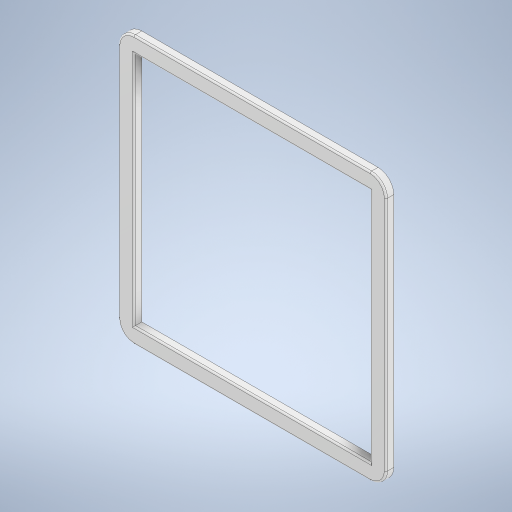
# Autodesk Inventor part: frame_inner
Saved by Autodesk Inventor 2023 (Build 270158000, 158)
## iProperties
Created: 2022-11-05
Part Number: frame_inner
Material: Acetalharz, Weiß
Document SubType Name: Modeling
Designer: RubenStein
Density: 1.425 g/cm^3
Appearance: Glatt - Weiß
Mass: 44.9884 g
Surface Area: 189.425 cm^2
Volume: 31.5708 cm^3
Author: RubenStein
Autodesk Inventor part; units mm, degrees
ref_plane "YZ Plane" through (0, 0, 0) normal (1, 0, 0) x (0, 1, 0)
ref_plane "XZ Plane" through (0, 0, 0) normal (0, 1, 0) x (-1, 0, 0)
ref_plane "XY Plane" through (0, 0, 0) normal (0, 0, 1) x (1, 0, 0)
sketch "Skizze1" plane through (0, 0, 0) normal (0, 0, 1) x (1, 0, 0)
  line L0 (0, 0) -> (170, 0)
  line L1 (170, 0) -> (170, 170)
  line L2 (170, 170) -> (0, 170)
  line L3 (0, 170) -> (0, 0)
  line L4 (10, 10) -> (160, 10)
  line L5 (160, 10) -> (160, 160)
  line L6 (160, 160) -> (10, 160)
  line L7 (10, 160) -> (10, 10)
  dimension "d0" = 170
  dimension "d1" = 10
  dimension "d2" = 10
  dimension "d3" = 150
  constraints: 16 end point, 4 parallel, 4 perpendicular, 2 horizontal
  measures "d0" distance of L1.end L2.end
  measures "d1" distance between parallel lines of L0 L4
  measures "d2" distance between parallel lines of L3 L7
  measures "d3" distance of L4.start L4.end
extrude "Extrusion1" add sketch "Skizze1" along normal blind 5
fillet "Rundung1" radius 10 4 edges at (170, 170, 2.5) (170, 0, 2.5) (0, 0, 2.5) (0, 170, 2.5)
fillet "Rundung2" radius 1 12 edges at (85, 160, 5) (10, 85, 5) (85, 10, 5) (160, 85, 5) (167.0711, 167.0711, 5) (85, 170, 5) (2.9289, 167.0711, 5) (0, 85, 5) (2.9289, 2.9289, 5) (85, 0, 5) (167.0711, 2.9289, 5) (170, 85, 5)
equation "\"d2\" = d1"
